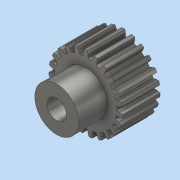
# Autodesk Inventor part: largeIdlerPinion
Saved by Autodesk Inventor 2017 (Build 210142000, 142)
## iProperties
Created: 2016-11-30
Part Number: largeIdlerPinion
Material: Steel, Carbon
Document SubType Name: Modeling
Designer: techn
Density: 7.85 g/cm^3
Appearance: Semi-Polished
Author: techn
Comments: A pinion gear i already own of the 20 to 24 tooth variety - adjust mesh in ballast section based on the axle pitch
Autodesk Inventor part; units mm, degrees
ref_plane "YZ Plane" through (0, 0, 0) normal (1, 0, 0) x (0, 1, 0)
ref_plane "XZ Plane" through (0, 0, 0) normal (0, 1, 0) x (-1, 0, 0)
ref_plane "XY Plane" through (0, 0, 0) normal (0, 0, 1) x (1, 0, 0)
sketch "Sketch1" plane through (0, 0, 0) normal (0, 0, 1) x (1, 0, 0)
  circle A0 centre (0, 0) radius 5.969
  dimension "d0" = 11.938
  constraints: 1 centre point, 1 coincident
  measures "d0" diameter of A0
extrude "Extrusion1" add sketch "Sketch1" along normal blind 6.096
sketch "Sketch2" plane through (0, 0, 6.096) normal (0, 0, 1) x (1, 0, 0)
  circle A0 centre (0, 0) radius 3.556
  dimension "d3" = 7.112
  constraints: 1 centre point, 1 coincident
  measures "d3" diameter of A0
extrude "Extrusion2" add sketch "Sketch2" along normal blind 4.699
sketch "Sketch3" plane through (0, 0, 10.795) normal (0, 0, 1) x (1, 0, 0)
  circle A0 centre (0, 0) radius 1.5875
  dimension "d6" = 3.175
  constraints: 1 centre point, 1 coincident
  measures "d6" diameter of A0
extrude "Extrusion3" cut sketch "Sketch3" against normal blind 25.4
sketch "Sketch4" plane through (0, 0, 0) normal (0, 0, -1) x (-1, 0, 0)
  circle A0 centre (0, 0) radius 5.0173
  line L0 (0.3683, 5.0038) -> (0.3683, 5.52)
  line L1 (0.3683, 5.52) -> (0.2667, 5.969)
  line L2 (0.2667, 5.969) -> (-0.2667, 5.969)
  line L3 (-0.2667, 5.969) -> (-0.3683, 5.52)
  line L4 (-0.3683, 5.52) -> (-0.3683, 5.0038)
  line L5 (-0.3683, 5.0038) -> (0.3683, 5.0038)
  circle A1 centre (0, 0) radius 6.7926
  line L6 (-1.8672, 5.6757) -> (-1.8439, 5.2159)
  line L7 (-1.3536, 5.8196) -> (-1.8672, 5.6757)
  line L8 (-1.1346, 5.4146) -> (-1.3536, 5.8196)
  line L9 (-0.9954, 4.9176) -> (-1.1346, 5.4146)
  line L10 (-1.7047, 4.7189) -> (-0.9954, 4.9176)
  line L11 (-1.8439, 5.2159) -> (-1.7047, 4.7189)
  line L12 (-3.3293, 4.9615) -> (-3.1828, 4.525)
  line L13 (-2.8735, 5.2386) -> (-3.3293, 4.9615)
  line L14 (-2.5534, 4.9077) -> (-2.8735, 5.2386)
  line L15 (-2.2852, 4.4667) -> (-2.5534, 4.9077)
  line L16 (-2.9146, 4.084) -> (-2.2852, 4.4667)
  line L17 (-3.1828, 4.525) -> (-2.9146, 4.084)
  line L18 (-4.5444, 3.8792) -> (-4.2856, 3.4985)
  line L19 (-4.1803, 4.2691) -> (-4.5444, 3.8792)
  line L20 (-3.7828, 4.0368) -> (-4.1803, 4.2691)
  line L21 (-3.4056, 3.6845) -> (-3.7828, 4.0368)
  line L22 (-3.9083, 3.1462) -> (-3.4056, 3.6845)
  line L23 (-4.2856, 3.4985) -> (-3.9083, 3.1462)
  line L24 (-5.4225, 2.5093) -> (-5.0705, 2.2125)
  line L25 (-5.1771, 2.9829) -> (-5.4225, 2.5093)
  line L26 (-4.7317, 2.8666) -> (-5.1771, 2.9829)
  line L27 (-4.2734, 2.6291) -> (-4.7317, 2.8666)
  line L28 (-4.6122, 1.9751) -> (-4.2734, 2.6291)
  line L29 (-5.0705, 2.2125) -> (-4.6122, 1.9751)
  line L30 (-5.8984, 0.9533) -> (-5.4794, 0.7625)
  line L31 (-5.7899, 1.4756) -> (-5.8984, 0.9533)
  line L32 (-5.3296, 1.4837) -> (-5.7899, 1.4756)
  line L33 (-4.8242, 1.3786) -> (-5.3296, 1.4837)
  line L34 (-4.9741, 0.6575) -> (-4.8242, 1.3786)
  line L35 (-5.4794, 0.7625) -> (-4.9741, 0.6575)
  line L36 (-5.9369, -0.6734) -> (-5.482, -0.7441)
  line L37 (-5.9733, -0.1413) -> (-5.9369, -0.6734)
  line L38 (-5.5322, -0.0093) -> (-5.9733, -0.1413)
  line L39 (-5.0173, 0.026) -> (-5.5322, -0.0093)
  line L40 (-4.967, -0.7089) -> (-5.0173, 0.026)
  line L41 (-5.482, -0.7441) -> (-4.967, -0.7089)
  line L42 (-5.535, -2.2502) -> (-5.0779, -2.1956)
  line L43 (-5.7137, -1.7476) -> (-5.535, -2.2502)
  line L44 (-5.3246, -1.5015) -> (-5.7137, -1.7476)
  line L45 (-4.8382, -1.3286) -> (-5.3246, -1.5015)
  line L46 (-4.5915, -2.0227) -> (-4.8382, -1.3286)
  line L47 (-5.0779, -2.1956) -> (-4.5915, -2.0227)
  line L48 (-4.7227, -3.6601) -> (-4.2973, -3.4841)
  line L49 (-5.0303, -3.2243) -> (-4.7227, -3.6601)
  line L50 (-4.722, -2.8824) -> (-5.0303, -3.2243)
  line L51 (-4.3003, -2.5847) -> (-4.722, -2.8824)
  line L52 (-3.8756, -3.1865) -> (-4.3003, -2.5847)
  line L53 (-4.2973, -3.4841) -> (-3.8756, -3.1865)
  line L54 (-3.5601, -4.7985) -> (-3.1979, -4.5143)
  line L55 (-3.9738, -4.4619) -> (-3.5601, -4.7985)
  line L56 (-3.7693, -4.0495) -> (-3.9738, -4.4619)
  line L57 (-3.4435, -3.6491) -> (-3.7693, -4.0495)
  line L58 (-2.8721, -4.1139) -> (-3.4435, -3.6491)
  line L59 (-3.1979, -4.5143) -> (-2.8721, -4.1139)
  line L60 (-2.1334, -5.5811) -> (-1.8614, -5.2097)
  line L61 (-2.6227, -5.3686) -> (-2.1334, -5.5811)
  line L62 (-2.537, -4.9162) -> (-2.6227, -5.3686)
  line L63 (-2.3313, -4.4428) -> (-2.537, -4.9162)
  line L64 (-1.6557, -4.7363) -> (-2.3313, -4.4428)
  line L65 (-1.8614, -5.2097) -> (-1.6557, -4.7363)
  line L66 (-0.5486, -5.9497) -> (-0.3868, -5.5187)
  line L67 (-1.077, -5.8771) -> (-0.5486, -5.9497)
  line L68 (-1.1165, -5.4184) -> (-1.077, -5.8771)
  line L69 (-1.0462, -4.907) -> (-1.1165, -5.4184)
  line L70 (-0.3165, -5.0073) -> (-1.0462, -4.907)
  line L71 (-0.3868, -5.5187) -> (-0.3165, -5.0073)
  line L72 (1.077, -5.8771) -> (1.1165, -5.4184)
  line L73 (0.5486, -5.9497) -> (1.077, -5.8771)
  line L74 (0.3868, -5.5187) -> (0.5486, -5.9497)
  line L75 (0.3165, -5.0073) -> (0.3868, -5.5187)
  line L76 (1.0462, -4.907) -> (0.3165, -5.0073)
  line L77 (1.1165, -5.4184) -> (1.0462, -4.907)
  line L78 (2.6227, -5.3686) -> (2.537, -4.9162)
  line L79 (2.1334, -5.5811) -> (2.6227, -5.3686)
  line L80 (1.8614, -5.2097) -> (2.1334, -5.5811)
  line L81 (1.6557, -4.7363) -> (1.8614, -5.2097)
  line L82 (2.3313, -4.4428) -> (1.6557, -4.7363)
  line L83 (2.537, -4.9162) -> (2.3313, -4.4428)
  line L84 (3.9738, -4.4619) -> (3.7693, -4.0495)
  line L85 (3.5601, -4.7985) -> (3.9738, -4.4619)
  line L86 (3.1979, -4.5143) -> (3.5601, -4.7985)
  line L87 (2.8721, -4.1139) -> (3.1979, -4.5143)
  line L88 (3.4435, -3.6491) -> (2.8721, -4.1139)
  line L89 (3.7693, -4.0495) -> (3.4435, -3.6491)
  line L90 (5.0303, -3.2243) -> (4.722, -2.8824)
  line L91 (4.7227, -3.6601) -> (5.0303, -3.2243)
  line L92 (4.2973, -3.4841) -> (4.7227, -3.6601)
  line L93 (3.8756, -3.1865) -> (4.2973, -3.4841)
  line L94 (4.3003, -2.5847) -> (3.8756, -3.1865)
  line L95 (4.722, -2.8824) -> (4.3003, -2.5847)
  line L96 (5.7137, -1.7476) -> (5.3246, -1.5015)
  line L97 (5.535, -2.2502) -> (5.7137, -1.7476)
  line L98 (5.0779, -2.1956) -> (5.535, -2.2502)
  line L99 (4.5915, -2.0227) -> (5.0779, -2.1956)
  line L100 (4.8382, -1.3286) -> (4.5915, -2.0227)
  line L101 (5.3246, -1.5015) -> (4.8382, -1.3286)
  line L102 (5.9733, -0.1413) -> (5.5322, -0.0093)
  line L103 (5.9369, -0.6734) -> (5.9733, -0.1413)
  line L104 (5.482, -0.7441) -> (5.9369, -0.6734)
  line L105 (4.967, -0.7089) -> (5.482, -0.7441)
  line L106 (5.0173, 0.026) -> (4.967, -0.7089)
  line L107 (5.5322, -0.0093) -> (5.0173, 0.026)
  line L108 (5.7899, 1.4756) -> (5.3296, 1.4837)
  line L109 (5.8984, 0.9533) -> (5.7899, 1.4756)
  line L110 (5.4794, 0.7625) -> (5.8984, 0.9533)
  line L111 (4.9741, 0.6575) -> (5.4794, 0.7625)
  line L112 (4.8242, 1.3786) -> (4.9741, 0.6575)
  line L113 (5.3296, 1.4837) -> (4.8242, 1.3786)
  line L114 (5.1771, 2.9829) -> (4.7317, 2.8666)
  line L115 (5.4225, 2.5093) -> (5.1771, 2.9829)
  line L116 (5.0705, 2.2125) -> (5.4225, 2.5093)
  line L117 (4.6122, 1.9751) -> (5.0705, 2.2125)
  line L118 (4.2734, 2.6291) -> (4.6122, 1.9751)
  line L119 (4.7317, 2.8666) -> (4.2734, 2.6291)
  line L120 (4.1803, 4.2691) -> (3.7828, 4.0368)
  line L121 (4.5444, 3.8792) -> (4.1803, 4.2691)
  line L122 (4.2856, 3.4985) -> (4.5444, 3.8792)
  line L123 (3.9083, 3.1462) -> (4.2856, 3.4985)
  line L124 (3.4056, 3.6845) -> (3.9083, 3.1462)
  line L125 (3.7828, 4.0368) -> (3.4056, 3.6845)
  line L126 (2.8735, 5.2386) -> (2.5534, 4.9077)
  line L127 (3.3293, 4.9615) -> (2.8735, 5.2386)
  line L128 (3.1828, 4.525) -> (3.3293, 4.9615)
  line L129 (2.9146, 4.084) -> (3.1828, 4.525)
  line L130 (2.2852, 4.4667) -> (2.9146, 4.084)
  line L131 (2.5534, 4.9077) -> (2.2852, 4.4667)
  line L132 (1.3536, 5.8196) -> (1.1346, 5.4146)
  line L133 (1.8672, 5.6757) -> (1.3536, 5.8196)
  line L134 (1.8439, 5.2159) -> (1.8672, 5.6757)
  line L135 (1.7047, 4.7189) -> (1.8439, 5.2159)
  line L136 (0.9954, 4.9176) -> (1.7047, 4.7189)
  line L137 (1.1346, 5.4146) -> (0.9954, 4.9176)
  dimension "d9" = 0.9652
  dimension "d10" = 0.5162
  dimension "d11" = 0.7366
  dimension "d12" = 0.5334
  dimension "d13" = 5.969
  dimension "d16" = 360
  constraints: 276 end point, 2 centre point, 2 coincident, 2 equal length, 2 point on circle, 1 horizontal, 1 parallel, 1 perpendicular, 1 vertical, 277 other
  measures "d9" distance between parallel lines of L5 L2
  measures "d10" distance of L0.start L0.end
  measures "d11" distance between parallel lines of L4 L0
  measures "d12" distance of L1.end L2.end
  measures "d13" distance from line of point (0, 0) L2
extrude "Extrusion4" cut sketch "Sketch4" against normal up to surface (6.096 mm away)
body "Solid1"
